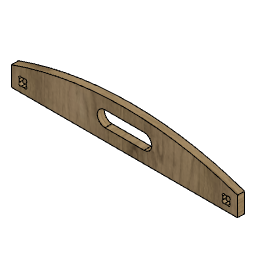
efra_saeti (Autodesk Fusion 360 design; units mm, degrees)
Autodesk Fusion 360 part; units mm, degrees
sketch "Sketch1" plane through (0, 0, 0) normal (0, 1, 0) x (1, 0, 0)
  line L0 (0, 0) -> (580, 0)
  line L1 (580, 0) -> (580, -50)
  line L2 (0, -50) -> (0, 0)
  arc A0 (0, -50) -> (580, -50) centre (290, 766) ccw
  line L3 (340, -70) -> (240, -70)
  line L4 (220, -50) -> (220, -50)
  line L5 (240, -30) -> (340, -30)
  line L6 (360, -50) -> (360, -50)
  arc A1 (220, -50) -> (240, -70) centre (240, -50) ccw
  arc A2 (240, -30) -> (220, -50) centre (240, -50) ccw
  arc A3 (340, -70) -> (360, -50) centre (340, -50) ccw
  arc A4 (360, -50) -> (340, -30) centre (340, -50) ccw
  point P0 (290, -50)
  dimension "d4" = 580
  dimension "d5" = 50
  dimension "d49" = 20
  constraint horizontal L0
  constraint vertical L1
  constraint vertical L2
  constraint coincident L0.start L2.end
  constraint horizontal L3
  constraint parallel L3 L5
  constraint tangent L3 A1
  constraint tangent L5 A2
  constraint equal A1 A2
  constraint tangent L3 A3
  constraint equal A1 A3
  constraint tangent L5 A4
  constraint equal A1 A4
  measures "d4" distance of L0.start L0.end
  measures "d5" distance of L0.start L2.start
  measures "d49" radius of A1
extrude "Extrude1" add sketch "Sketch1" along normal blind 18
sketch "Sketch2" plane through (0, 0, 0) normal (0, -1, 0) x (1, 0, 0)
  line L0 (340, 30) -> (240, 30)
  line L1 (240, 70) -> (340, 70)
  line L2 (0, 50) -> (0, 0)
  line L3 (0, 0) -> (580, 0)
  line L4 (580, 0) -> (580, 50)
  arc A0 (580, 50) -> (0, 50) centre (290, -766) ccw
  line L5 (25.3517, 35) -> (32.6483, 35)
  line L6 (38, 29.0536) -> (38, 20.9464)
  line L7 (32.6483, 15) -> (25.3517, 15)
  line L8 (20, 20.9464) -> (20, 29.0536)
  line L9 (542, 20.9464) -> (542, 29.0536)
  line L10 (547.3517, 35) -> (554.6483, 35)
  line L11 (560, 29.0536) -> (560, 20.9464)
  line L12 (554.6483, 15) -> (547.3517, 15)
  line L13 (542, 20.9464) -> (542, 29.0536)
  line L14 (554.6483, 15) -> (547.3517, 15)
  line L15 (547.3517, 35) -> (554.6483, 35)
  line L16 (560, 29.0536) -> (560, 20.9464)
  arc A1 (340, 30) -> (340, 70) centre (340, 50) ccw
  arc A2 (240, 70) -> (240, 30) centre (240, 50) ccw
  arc A3 (25.3517, 35) -> (20, 29.0536) centre (22.6759, 32.0268) ccw
  arc A4 (38, 29.0536) -> (32.6483, 35) centre (35.3241, 32.0268) ccw
  arc A5 (32.6483, 15) -> (38, 20.9464) centre (35.3241, 17.9732) ccw
  line L17 (25.3517, 20.9464) -> (20, 15)
  arc A6 (20, 20.9464) -> (25.3517, 15) centre (22.6759, 17.9732) ccw
  arc A7 (547.3517, 35) -> (542, 29.0536) centre (544.6759, 32.0268) ccw
  arc A8 (560, 29.0536) -> (554.6483, 35) centre (557.3241, 32.0268) ccw
  arc A9 (554.6483, 15) -> (560, 20.9464) centre (557.3241, 17.9732) ccw
  arc A10 (542, 20.9464) -> (547.3517, 15) centre (544.6759, 17.9732) ccw
  arc A11 (547.3517, 35) -> (542, 29.0536) centre (544.6759, 32.0268) ccw
  arc A12 (542, 20.9464) -> (547.3517, 15) centre (544.6759, 17.9732) ccw
  arc A13 (554.6483, 15) -> (560, 20.9464) centre (557.3241, 17.9732) ccw
  arc A14 (560, 29.0536) -> (554.6483, 35) centre (557.3241, 32.0268) ccw
  dimension "d25" = 8
  dimension "d26" = 8
  dimension "d27" = 8
  dimension "d28" = 8
  dimension "d33" = 8
  dimension "d34" = 8
  dimension "d35" = 8
  dimension "d36" = 8
  dimension "d45" = 8
  dimension "d46" = 8
  dimension "d47" = 8
  dimension "d48" = 8
  constraint horizontal L5
  constraint vertical L6
  constraint horizontal L7
  constraint vertical L8
  constraint coincident L17.end A6
  constraint horizontal L10
  constraint vertical L11
  constraint horizontal L12
  constraint vertical L9
  constraint horizontal L15
  constraint vertical L16
  constraint horizontal L14
  constraint vertical L13
  measures "d25" diameter of A3
  measures "d26" diameter of A4
  measures "d27" diameter of A5
  measures "d28" diameter of A6
  measures "d33" diameter of A11
  measures "d34" diameter of A8
  measures "d35" diameter of A9
  measures "d36" diameter of A12
  measures "d45" diameter of A7
  measures "d46" diameter of A14
  measures "d47" diameter of A13
  measures "d48" diameter of A10
extrude "Extrude3" cut sketch "Sketch2" against normal blind 10 contours L5 L6 L7 L8 A3 A4 A5 A6 | L9 L10 L11 L12 L13 L14 L15 L16 A7 A8 A9 A10 A11 A12 A13 A14
equation "breidd_bak = 50 mm"
equation "t_bak = 18 mm"
equation "lengd_bak = 580 mm"
equation "d4 = lengd_bak"
equation "d5 = breidd_bak"
equation "dog_r = 8 mm"
equation "d25 = dog_r"
equation "d26 = dog_r"
equation "d27 = dog_r"
equation "d28 = dog_r"
equation "d33 = dog_r"
equation "d34 = dog_r"
equation "d35 = dog_r"
equation "d36 = dog_r"
equation "d45 = dog_r"
equation "d46 = dog_r"
equation "d47 = dog_r"
equation "d48 = dog_r"
